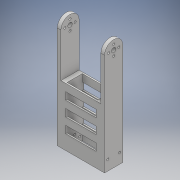
# Autodesk Inventor part: arm_1
Saved by Autodesk Inventor 2018 (Build 220112000, 112)
## iProperties
Created: 2018-02-05
Part Number: arm_1
Material: Genérico
Document SubType Name: Modeling
Designer: se_ma
Density: 1 g/cm^3
Appearance: Valor por defecto
Author: se_ma
Autodesk Inventor part; units mm, degrees
ref_plane "YZ Plane" through (0, 0, 0) normal (1, 0, 0) x (0, 1, 0)
ref_plane "XZ Plane" through (0, 0, 0) normal (0, 1, 0) x (-1, 0, 0)
ref_plane "XY Plane" through (0, 0, 0) normal (0, 0, 1) x (1, 0, 0)
sketch "Boceto1" plane through (0, 0, 0) normal (0, 1, 0) x (-1, 0, 0)
  line L0 (0, 0) -> (60, 0)
  line L1 (60, 0) -> (60, -80)
  line L2 (60, -80) -> (0, -80)
  line L3 (0, -80) -> (0, 0)
  dimension "d0" = 60
  dimension "d1" = 80
  constraints: 8 end point, 2 parallel, 1 horizontal, 1 perpendicular
  measures "d0" distance of L1.end L2.end
  measures "d1" distance of L0.end L1.end
extrude "Extrusión1" add sketch "Boceto1" along normal blind 25
sketch "Boceto2" plane through (-60, 0, 0) normal (0, 0, 1) x (1, 0, 0)
  line L0 (0, 25) -> (60, 25) projected
  line L1 (30, 25) -> (30, 23)
  line L2 (60, 0) -> (0, 0) projected
  line L3 (30, 0) -> (30, 2)
  line L4 (0, 0) -> (0, 25) projected
  line L5 (60, 0) -> (60, 25) projected
  line L6 (30, 23) -> (9, 23)
  line L7 (9, 2) -> (30, 2)
  line L8 (30, 23) -> (51, 23)
  line L9 (51, 2) -> (30, 2)
  line L10 (9, 23) -> (9, 19.5)
  line L11 (9, 2) -> (9, 5.5)
  arc A0 (9, 19.5) -> (1, 12.5) centre (7.9996, 12.5719) ccw
  arc A1 (1, 12.5) -> (9, 5.5) centre (7.9996, 12.4281) ccw
  line L12 (51, 23) -> (51, 19.5)
  line L13 (51, 2) -> (51, 5.5)
  arc A2 (59, 12.5) -> (51, 19.5) centre (52.0004, 12.5719) ccw
  arc A3 (51, 5.5) -> (59, 12.5) centre (52.0004, 12.4281) ccw
  dimension "d4" = 2
  dimension "d5" = 2
  dimension "d7" = 21
  dimension "d12" = 3.5
  dimension "d13" = 3.5
  dimension "d15" = 7
  dimension "d16" = 7
  dimension "d17" = 3.5
  dimension "d18" = 3.5
  dimension "d19" = 7
  dimension "d20" = 7
  constraints: 20 end point, 8 point on circle, 5 vertical, 4 centre point, 2 midpoint, 2 point on line, 1 horizontal
  measures "d4" distance of L1.start L1.end
  measures "d5" distance of L3.start L3.end
  measures "d7" distance of L1.end L8.end
  measures "d12" distance of L6.end L10.end
  measures "d13" distance of L7.start L11.end
  measures "d15" radius of A0
  measures "d16" radius of A1
  measures "d17" distance of L8.end L12.end
  measures "d18" distance of L9.start L13.end
  measures "d19" radius of A2
  measures "d20" radius of A3
extrude "Extrusión2" cut sketch "Boceto2" against normal blind 80 contours L8 L12 A2 A3 L13 L9 L7 L11 A1 A0 L10 L6
move faces "Desplazar1" translate (-1, 0, 0) faces at (-60, 8.3333, -26.6667)
move faces "Desplazar2" translate (1, 0, 0) faces at (0, 8.3333, -53.3333)
sketch "Boceto3" plane through (1, 0, 0) normal (1, 0, 0) x (0, 0, -1)
  line L0 (0, 0) -> (80, 0) projected
  line L1 (80, 0) -> (80, 25) projected
  line L2 (80, 0) -> (80, 25)
  line L3 (80, 25) -> (-60, 25)
  circle A0 centre (-60, 19.5) radius 1.5
  circle A1 centre (-67, 12.5) radius 1.5
  circle A2 centre (-60, 5.5) radius 1.5
  circle A3 centre (-53, 12.5) radius 1.5
  circle A4 centre (-60, 12.5) radius 3
  line L4 (80, 0) -> (-60, 0)
  arc A5 (-60, 25) -> (-60, 0) centre (-60, 12.5) ccw
  dimension "d29" = 25
  dimension "d30" = 140
  dimension "d35" = 3
  dimension "d36" = 3
  dimension "d37" = 3
  dimension "d38" = 3
  dimension "d39" = 6
  constraints: 6 centre point, 6 end point, 2 point on circle, 1 coincident, 1 horizontal, 1 perpendicular, 1 vertical
  measures "d29" distance of L0.end L1.end
  measures "d30" distance of L1.end L3.end
  measures "d35" diameter of A0
  measures "d36" diameter of A1
  measures "d37" diameter of A2
  measures "d38" diameter of A3
  measures "d39" diameter of A4
extrude "Extrusión3" add sketch "Boceto3" along normal blind 5
sketch "Boceto5" plane through (-61, 0, -80) normal (-1, 0, 0) x (0, 0, 1)
  line L0 (0, 0) -> (0, 25) projected
  line L1 (0, 0) -> (0, 25)
  line L2 (0, 25) -> (140, 25)
  line L3 (0, 0) -> (140, 0)
  circle A0 centre (140, 12.5) radius 3 projected
  circle A1 centre (140, 12.5) radius 3
  circle A2 centre (140, 19.5) radius 1.5
  circle A3 centre (133, 12.5) radius 1.5
  circle A4 centre (147, 12.5) radius 1.5
  circle A5 centre (140, 5.5) radius 1.5
  arc A6 (140, 0) -> (140, 25) centre (140, 12.5) ccw
  point P0 (80, 0)
  dimension "d52" = 3
  dimension "d53" = 3
  dimension "d54" = 3
  dimension "d55" = 3
  constraints: 6 centre point, 6 end point, 2 coincident, 2 point on circle, 1 horizontal, 1 perpendicular, 1 vertical
  measures "d52" diameter of A2
  measures "d53" diameter of A3
  measures "d54" diameter of A4
  measures "d55" diameter of A5
extrude "Extrusión4" add sketch "Boceto5" along normal blind 5
sketch "Boceto7" plane through (6, 0, -80) normal (0, 0, -1) x (-1, 0, 0)
  line L0 (57, 2) -> (15, 2) projected
  line L1 (57, 2) -> (65, 2)
  line L2 (65, 2) -> (65, 23)
  line L3 (57, 23) -> (15, 23) projected
  line L4 (65, 23) -> (57, 23)
  line L5 (57, 23) -> (57, 2)
  line L6 (15, 2) -> (7, 2)
  line L7 (7, 2) -> (7, 23)
  line L8 (7, 23) -> (15, 23)
  line L9 (15, 2) -> (15, 5.5) projected
  line L10 (15, 2) -> (15, 23)
  point P0 (6, 0)
  dimension "d60" = 8
  dimension "d61" = 21
  dimension "d62" = 8
  constraints: 16 end point, 5 perpendicular, 2 horizontal
  measures "d60" distance of L0.start L1.end
  measures "d61" distance of L1.end L2.end
  measures "d62" distance of L0.end L6.end
extrude "Extrusión5" add sketch "Boceto7" against normal blind 80 contours L5 L4 L2 L1 | L6 L7 L8 L10 L9
move faces "Desplazar3" translate (3.5, 0, 0) faces at (-61, 12.5, 17.1667) (-66, 12.5, -36.1667)
move faces "Desplazar4" translate (-3.5, 0, 0) faces at (1, 12.5, 17.1667) (6, 12.5, -36.1667)
sketch "Boceto8" plane through (-62.5, 12.5, 60) normal (-1, 0, 0) x (0, 0, 1)
  line L0 (-140, 0) -> (-127, 0)
  circle A0 centre (-127, 0) radius 1.5
  line L1 (-140, -12.5) -> (-140, -7)
  line L2 (-140, -7) -> (-133, -7)
  line L3 (-140, 12.5) -> (-140, 7)
  line L4 (-140, 12.5) -> (-140, -12.5) projected
  line L5 (-140, 7) -> (-133, 7)
  circle A1 centre (-133, -7) radius 1.5
  circle A2 centre (-133, 7) radius 1.5
  point P0 (-60, -12.5)
  dimension "d75" = 13
  dimension "d77" = 3
  dimension "d79" = 5.5
  dimension "d80" = 5.5
  dimension "d81" = 7
  dimension "d82" = 3
  dimension "d83" = 3
  constraints: 10 end point, 3 centre point, 3 coincident, 2 perpendicular, 1 horizontal, 1 point on line
  measures "d75" distance of L0.start L0.end
  measures "d77" diameter of A0
  measures "d79" distance of L1.start L1.end
  measures "d80" distance of L3.start L3.end
  measures "d81" distance of L3.end L5.end
  measures "d82" diameter of A1
  measures "d83" diameter of A2
extrude "Extrusión6" cut sketch "Boceto8" against normal blind 11.5
sketch "Boceto9" plane through (2.5, 12.5, 60) normal (1, 0, 0) x (0, 0, -1)
  line L0 (140, 12.5) -> (140, -12.5) projected
  line L1 (140, 12.5) -> (140, 8)
  line L2 (140, -12.5) -> (140, -8)
  line L3 (140, 10.5) -> (140, -10.5) projected
  line L4 (140, 8) -> (126, 8)
  line L5 (60, 10.5) -> (140, 10.5) projected
  line L6 (140, 8) -> (154, 8) construction
  line L7 (140, -8) -> (126, -8)
  line L8 (60, -0.1437) -> (125.5069, -0.1437) projected
  line L9 (140, -8) -> (154, -8) construction
  circle A0 centre (126, 8) radius 1.5
  circle A1 centre (126, -8) radius 1.5
  point P0 (60, -12.5)
  dimension "d86" = 4.5
  dimension "d87" = 4.5
  dimension "d88" = 14
  dimension "d89" = 180
  dimension "d90" = 14
  dimension "d91" = 180
  dimension "d92" = 3
  dimension "d93" = 3
  constraints: 12 end point, 2 centre point, 2 coincident, 2 collinear, 2 horizontal, 2 parallel, 2 point on line
  measures "d86" distance of L0.start L1.end
  measures "d87" distance of L0.end L2.end
  measures "d88" distance of L1.end L4.end
  measures "d89" angle of L4 L6
  measures "d90" distance of L2.end L7.end
  measures "d91" angle of L7 L9
  measures "d92" diameter of A0
  measures "d93" diameter of A1
extrude "Extrusión7" cut sketch "Boceto9" against normal blind 11.5
sketch "Boceto10" plane through (0, 25, 0) normal (0, 1, 0) x (1, 0, 0)
  line L0 (-62.5, -60) -> (-62.5, 80) projected
  line L1 (-51, 80) -> (-51, 0)
  line L2 (-9, 80) -> (-9, 0)
  line L3 (-57.5, 0) -> (-2.5, 0) projected
  line L4 (-51, 0) -> (-51, 10)
  line L5 (-9, 0) -> (-9, 80) projected
  line L6 (-9, 0) -> (-9, 80) projected
  line L7 (-51, 20) -> (-51, 30)
  line L8 (-51, 30) -> (-51, 40)
  line L9 (-51, 40) -> (-51, 50)
  line L10 (-51, 50) -> (-51, 60)
  line L11 (-51, 60) -> (-9, 60)
  line L12 (-51, 60) -> (-51, 70)
  line L13 (-51, 10) -> (-9, 10)
  line L14 (-51, 20) -> (-9, 20)
  line L15 (-51, 30) -> (-9, 30)
  line L16 (-51, 40) -> (-9, 40)
  line L17 (-51, 50) -> (-9, 50)
  point P0 (0, 0)
  point P1 (2.5, 80)
  dimension "d96" = 10
  dimension "d97" = 10
  dimension "d98" = 10
  dimension "d99" = 10
  dimension "d100" = 10
  dimension "d101" = 10
  constraints: 26 end point, 6 point on line, 5 perpendicular, 1 midpoint, 10 other
  measures "d96" distance of L4.end L7.start
  measures "d97" distance of L7.start L7.end
  measures "d98" distance of L7.end L8.end
  measures "d99" distance of L8.end L9.end
  measures "d100" distance of L9.end L10.end
  measures "d101" distance of L10.end L12.end
extrude "Extrusión8" cut sketch "Boceto10" against normal blind 25 contours L11 L2 L17 L1 | L16 L2 L15 L1 | L14 L2 L13 L1
